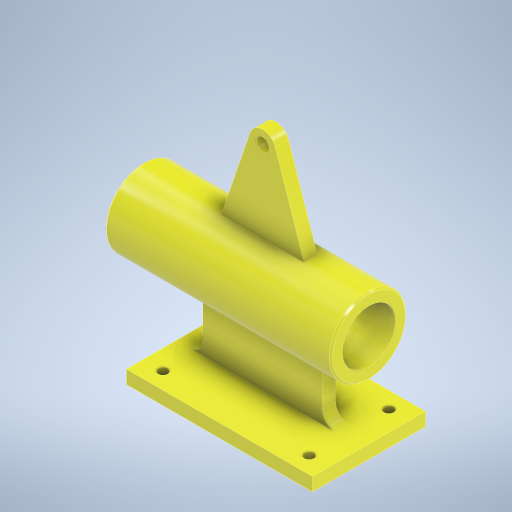
# Autodesk Inventor part: 1 HUDSON-8-28A-TDR HAND PUMP BASE BODY
Saved by Autodesk Inventor 2024.2 (Build 282272000, 272)
## iProperties
Created: 2024-11-02
Part Number: 1 HUDSON-8-28A-TDR HAND PUMP BASE BODY
Material: Genérico
Document SubType Name: Modeling
Designer: brene
Density: 1 g/cm^3
Appearance: Amarillo
Author: brene
Autodesk Inventor part; units mm, degrees
ref_plane "YZ Plane" through (0, 0, 0) normal (1, 0, 0) x (0, 1, 0)
ref_plane "XZ Plane" through (0, 0, 0) normal (0, 1, 0) x (-1, 0, 0)
ref_plane "XY Plane" through (0, 0, 0) normal (0, 0, 1) x (1, 0, 0)
sketch "Boceto1" plane through (0, 0, 0) normal (0, 0, 1) x (1, 0, 0)
  line L0 (0, 31.2124) -> (0, -31.2124) construction
  line L1 (-43.2332, 0) -> (43.2332, 0)
  line L2 (-34, 11.5) -> (34, 11.5)
  line L3 (34, -11.5) -> (-34, -11.5)
  line L4 (-34, 8) -> (34, 8)
  arc A0 (7.7895, 37.2804) -> (0.2105, 37.2804) centre (4, 36) ccw
  circle A1 centre (4, 36) radius 2
  line L5 (0.4937, 38.1188) -> (-8.5, 11.5)
  line L6 (7.7895, 37.2804) -> (16.5, 11.5)
  line L7 (-14, -11.5) -> (-14, -24)
  line L8 (22, -11.5) -> (22, -24)
  line L9 (-14, -28) -> (22, -28)
  line L10 (-22, -28) -> (34, -28)
  line L11 (-22, -28) -> (-22, -32)
  line L12 (-22, -32) -> (34, -32)
  line L13 (34, -32) -> (34, -28)
  arc A2 (-18, -28) -> (-14, -24) centre (-18, -24) ccw
  arc A3 (22, -24) -> (26, -28) centre (26, -24) ccw
  line L14 (4, 46.9888) -> (4, 11.5)
  line L15 (-34, 11.5) -> (-34, 8)
  line L16 (34, 11.5) -> (34, 8)
  point P0 (0, 0)
  point P1 (0, 0)
  point P2 (0, 11.5)
  point P3 (22, -28)
  dimension "d0" = 23
  dimension "d1" = 68
  dimension "d2" = 23
  dimension "d3" = 16
  dimension "d4" = 30
  dimension "d5" = 8
  dimension "d6" = 4
  dimension "d10" = 24.5
  dimension "d11" = 12
  dimension "d12" = 20
  dimension "d13" = 16.5
  dimension "d14" = 16.5
  dimension "d15" = 56
  dimension "d16" = 0
  dimension "d17" = 4
  dimension "d20" = 4
  dimension "d24" = 56
  dimension "d27" = 9.322
  dimension "d28" = 12.5
  dimension "d29" = 12.5
  dimension "d30" = 30
  dimension "d31" = 9.2332
  dimension "d32" = 0
  dimension "d33" = 0.4825
  dimension "d34" = 33.5063
  dimension "d35" = 68
  constraints: 34 end point, 11 point on line, 8 tangent, 6 point on circle, 4 centre point, 4 horizontal, 4 vertical, 3 coincident, 3 midpoint, 3 perpendicular, 1 equal radius
  measures "d0" diameter of L2 L1
  measures "d1" distance of L2.start L2.end
  measures "d2" distance between parallel lines of L3 L2
  measures "d3" diameter of L4 L1
  measures "d4" horizontal distance of L2.end point (4, 36)
  measures "d5" diameter of A0
  measures "d6" diameter of A1
  measures "d10" vertical distance of L2.end A0.centre
  measures "d11" distance from line of L8 L3.start
  measures "d12" distance from line of L3.end L7
  measures "d13" distance of L7.start L9.start
  measures "d14" distance of L8.start L9.end
  measures "d15" distance of L10.start L10.end
  measures "d16" horizontal distance of L3.start L10.end
  measures "d17" distance of L10.start L11.end
  measures "d20" radius of A3
  measures "d24" diameter of L10 L1
  measures "d27" distance from line of L0.start L6
  measures "d28" distance from line of L6.end L14
  measures "d29" distance from line of L14 L5.end
  measures "d30" distance between parallel lines of L14 L13
  measures "d31" distance from line of L1.end L13
  measures "d32" distance from line of L4.end L13
  measures "d33" distance from line of L14.start L6
  measures "d34" distance from line of L5.start L13
  measures "d35" distance from line of L4.start L13
extrude "Extrusión1" add sketch "Boceto1" along normal blind 2 and the other way blind 2 contours L5 A0 L14 A1 L2 | L14 A1 A0 L6 L2
extrude "Extrusión2" add sketch "Boceto1" along normal blind 2 and the other way blind 2 contours L8 A3 L10 L9 A2 L7 L3
extrude "Extrusión3" add sketch "Boceto1" along normal blind 17 and the other way blind 17 contours L10 L13 L12 L11 L9
sketch "Boceto2" plane through (0, 0, 0) normal (0, 0, 1) x (1, 0, 0)
  line L0 (-8.5, 11.5) -> (16.5, 11.5) projected
  line L1 (16.5, 11.5) -> (-8.5, 11.5) projected
  line L2 (-8.5, 11.5) -> (16.5, 11.5) projected
  line L3 (16.5, 11.5) -> (-8.5, 11.5) projected
  line L4 (34, 11.5) -> (34, 8) projected
  line L5 (-34, 11.5) -> (34, 11.5) projected
  line L6 (-34, 8) -> (34, 8) projected
  line L7 (-34, 11.5) -> (-34, 8) projected
  line L8 (0, 31.2124) -> (0, -31.2124) construction
  line L9 (-43.2332, 0) -> (43.2332, 0) projected
  line L10 (-34, 11.5) -> (34, 11.5)
  line L11 (34, 11.5) -> (34, 8)
  line L12 (34, 8) -> (-34, 8)
  line L13 (-34, 8) -> (-34, 11.5)
  point P0 (0, 0)
  point P1 (0, 0)
  point P2 (0, 0)
  point P3 (0, 11.5)
  point P4 (-8.5, 11.5)
  point P5 (16.5, 11.5)
  point P6 (4, 11.5)
  dimension "d50" = 23
  constraints: 8 end point, 2 parallel, 1 horizontal, 1 perpendicular, 1 other
revolve "Revolución2" add sketch "Boceto2" angle 360 about axis through (-43.2332, 0, 0) along (1, 0, 0)
sketch "Boceto4" plane through (-22, -28, 17) normal (0, 1, 0) x (1, 0, 0)
  line L0 (56, 34) -> (56, 0) projected
  line L1 (56, 17) -> (0, 17)
  line L2 (0, 34) -> (0, 0) projected
  point P0 (22, 17)
  point P1 (50, 5)
  point P2 (50, 29)
  point P3 (6, 29)
  point P4 (6, 5)
  dimension "d54" = 6
  dimension "d55" = 12
  dimension "d56" = 6
  dimension "d57" = 12
  dimension "d58" = 6
  dimension "d59" = 12
  dimension "d60" = 6
  dimension "d61" = 12
  constraints: 2 end point, 2 midpoint
  measures "d54" horizontal distance of L0.end point (50, 5)
  measures "d55" vertical distance of L1.start point (50, 5)
  measures "d56" horizontal distance of L0.start point (50, 29)
  measures "d57" vertical distance of L1.start point (50, 29)
  measures "d58" horizontal distance of L2.start point (6, 29)
  measures "d59" vertical distance of L1.end point (6, 29)
  measures "d60" horizontal distance of L2.end point (6, 5)
  measures "d61" vertical distance of L1.end point (6, 5)
hole "Agujero1" at (28, -28, 12) at (28, -28, -12) at (-16, -28, -12) at (-16, -28, 12) direction (0, -1, 0) diameter 3 end through all
chamfer "Chaflán1" distance 0.5 angle 45 1 edges at (34, -11.5, 0)
chamfer "Chaflán2" distance 0.5 angle 45 1 edges at (-34, -11.5, 0)
equation "\"d14\" = d13"
equation "\"d56\" = d54"
equation "\"d57\" = d55"
equation "\"d58\" = d56"
equation "\"d59\" = d57"
equation "\"d60\" = d58"
equation "\"d61\" = d59"
